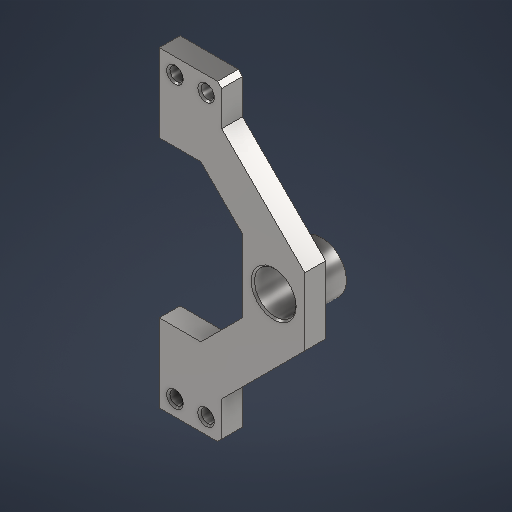
# Autodesk Inventor part: uchwyt-GM
Saved by Autodesk Inventor 2026.1 (Build 301233020, 233B)
## iProperties
Created: 2025-11-04
Part Number: uchwyt-GM
Material: Stainless Steel
Document SubType Name: Modeling
Designer: Jan
Density: 8 g/cm^3
Appearance: Semi-Polished
Author: Jan
Autodesk Inventor part; units mm, degrees
ref_plane "YZ Plane" through (0, 0, 0) normal (1, 0, 0) x (0, 1, 0)
ref_plane "XZ Plane" through (0, 0, 0) normal (0, 1, 0) x (-1, 0, 0)
sketch "Sketch1" plane through (0, 0, 0) normal (0, 0, 1) x (1, 0, 0)
  line L0 (-5.8474, 0) -> (5.8474, 0) construction
  line L1 (2.5, 18.75) -> (7.5, 18.75)
  line L2 (7.5, 18.75) -> (7.5, 37.5)
  line L3 (7.5, 37.5) -> (-7.5, 37.5)
  line L4 (-7.5, 37.5) -> (-7.5, 18.75)
  line L5 (-7.5, 18.75) -> (2.5, 18.75)
  circle A0 centre (3.75, 33.75) radius 1.6
  circle A1 centre (-3.75, 33.75) radius 1.6
  line L6 (2.5, -18.75) -> (7.5, -18.75)
  line L7 (7.5, -18.75) -> (7.5, -37.5)
  line L8 (7.5, -37.5) -> (-7.5, -37.5)
  line L9 (-7.5, -37.5) -> (-7.5, -18.75)
  line L10 (-7.5, -18.75) -> (2.5, -18.75)
  circle A2 centre (3.75, -33.75) radius 1.6
  circle A3 centre (-3.75, -33.75) radius 1.6
  line L11 (7.5, 28.125) -> (27.5, 8.125)
  line L12 (7.5, 28.125) -> (35.7843, 28.125) construction
  line L13 (2.5, 18.75) -> (12.5, 8.75)
  line L14 (12.5, 8.75) -> (12.5, 0)
  line L15 (27.5, 8.125) -> (27.5, 0)
  line L16 (7.5, -28.125) -> (27.5, -8.125)
  line L17 (2.5, -18.75) -> (12.5, -8.75)
  line L18 (12.5, -8.75) -> (12.5, 0)
  line L19 (27.5, -8.125) -> (27.5, 0)
  point P0 (0, 0)
  point P1 (0, 0)
  point P2 (2.5, -18.75)
  point P3 (2.5, -18.75)
  point P4 (2.5, 18.75)
  dimension "d2" = 15
  dimension "d3" = 18.75
  dimension "d4" = 7.5
  dimension "d5" = 3.2
  dimension "d6" = 3.2
  dimension "d7" = 3.75
  dimension "d8" = 3.75
  dimension "d9" = 7.5
  dimension "d10" = 18.75
  dimension "d20" = 45
  dimension "d21" = 20
  dimension "d31" = 20
  dimension "d32" = 10
  constraints: 40 end point, 11 symmetric about line, 5 perpendicular, 4 centre point, 4 point on line, 3 horizontal, 2 midpoint, 1 coincident, 1 equal length, 1 horizontal alignment, 1 parallel, 1 vertical, 2 other
  measures "d2" distance of L2.end L3.end
  measures "d3" distance between parallel lines of L3 L1
  measures "d4" distance from line of L4 point (0, 0)
  measures "d5" diameter of A0
  measures "d6" diameter of A1
  measures "d7" distance from line of L4 A1.centre
  measures "d8" horizontal distance of L3.end A1.centre
  measures "d9" distance of A1.centre A0.centre
  measures "d10" vertical distance of L1.end L0.end
  measures "d20" angle of L11 L12
  measures "d21" horizontal distance of L11.start L11.end
  measures "d31" distance between parallel lines of L4 L14
  measures "d32" horizontal distance of L13.end L13.start
ref_plane "Work Plane1" through (0, 0, 5) normal (0, 0, 1) x (1, 0, 0)
extrude "Extrusion3" add sketch "Sketch1" along normal blind 5
chamfer "Chamfer4" distance 0.4 angle 45 4 edges at (2.15, 33.75, 5) (-5.35, 33.75, 5) (2.15, -33.75, 5) (-5.35, -33.75, 5)
sketch "Sketch4" plane through (0, 0, 5) normal (0, 0, 1) x (1, 0, 0)
  circle A0 centre (20, 0) radius 5
  line L0 (27.5, -8.125) -> (27.5, 8.125) projected
  line L1 (12.5, 8.75) -> (12.5, -8.75) projected
  point P0 (0, 0)
  point P1 (12.5, 0)
  dimension "d40" = 10
  dimension "d41" = 15
  dimension "d42" = 7.5
  constraints: 1 centre point, 1 midpoint
  measures "d40" diameter of A0
  measures "d41" distance between parallel lines of L0 L1
  measures "d42" distance of A0.centre point (12.5, 0)
extrude "Extrusion5" cut sketch "Sketch4" against normal blind 5
chamfer "Chamfer5" distance 0.4 angle 45 1 edges at (15, 0, 5)
sketch "Sketch5" plane through (0, 0, 0) normal (0, 0, -1) x (-1, 0, 0)
  circle A0 centre (-20, 0) radius 5 projected
  circle A1 centre (-20, 0) radius 5
  circle A2 centre (-20, 0) radius 6
  point P0 (0, 0)
  dimension "d48" = 12
  constraints: 2 centre point, 2 coincident, 1 concentric
  measures "d48" diameter of A2
extrude "Extrusion6" add sketch "Sketch5" along normal blind 6.5
chamfer "Chamfer6" distance 1 angle 45 2 edges at (7.5, 37.5, 2.5) (7.5, -37.5, 2.5)
equation "\"d4\" = 0.5 * d2"
equation "\"d7\" = 0.25 * d2"
equation "\"d8\" = d7"
equation "\"d9\" = 0.5 * d2"
equation "\"d31\" = d21"
equation "\"d42\" = 0.5 * d41"
body "Solid1"
